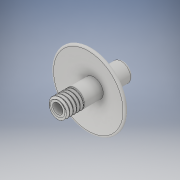
# Autodesk Inventor part: Kabelzugentlastung
Saved by Autodesk Inventor 2018.2 (Build 222227000, 227)
## iProperties
Created: 2018-01-25
Part Number: Kabelzugentlastung
Material: Generisch
Document SubType Name: Modeling
Designer: JochenAlt
Density: 1 g/cm^3
Appearance: Vorgabe
Author: JochenAlt
Autodesk Inventor part; units mm, degrees
ref_plane "YZ Plane" through (0, 0, 0) normal (1, 0, 0) x (0, 1, 0)
ref_plane "XZ Plane" through (0, 0, 0) normal (0, 1, 0) x (-1, 0, 0)
ref_plane "XY Plane" through (0, 0, 0) normal (0, 0, 1) x (1, 0, 0)
sketch "Skizze1" plane through (0, 0, 0) normal (0, 0, 1) x (1, 0, 0)
  line L0 (0, 93.8392) -> (0, -15.6399) construction
  line L1 (-4.2899, 0) -> (25.7393, 0) construction
  arc A0 (20.2057, 57.5563) -> (5.5, 60.7515) centre (0, 0) ccw
  arc A1 (20.09, 59.1831) -> (6.1759, 62.1941) centre (0, 0) ccw
  arc A2 (20.2057, 57.5563) -> (20.09, 59.1831) centre (20.5, 58.3948) ccw
  line L2 (5.5, 62.9404) -> (5.5, 76.6904)
  line L3 (4.25, 77.9404) -> (4.25, 77.9404)
  arc A3 (5.5, 62.9404) -> (6.1759, 62.1941) centre (6.25, 62.9404) ccw
  arc A4 (5.5, 76.6904) -> (4.25, 77.9404) centre (4.25, 76.6904) ccw
  arc A5 (4.25, 77.9404) -> (3, 76.6904) centre (4.25, 76.6904) ccw
  line L4 (5.5, 60.7515) -> (5.5, 39.7947)
  line L5 (3, 76.6904) -> (3, 62.9881)
  line L6 (3, 62.9881) -> (3, 39.7947)
  line L7 (3, 39.7947) -> (5.5, 39.7947)
  point P0 (20.0791, 59.1868)
  point P1 (17.7943, 58.3469)
  point P2 (20.1696, 59.2201)
  point P3 (20.1696, 59.2201)
  point P4 (5.5, 62.2575)
  dimension "d3" = 1.5
  dimension "d4" = 61
  dimension "d6" = 5.5
  dimension "d9" = 0.75
  dimension "d10" = 15
  dimension "d11" = 1.25
  dimension "d59" = 2.5
  dimension "d60" = 15
  constraints: 16 point on circle, 12 end point, 7 tangent, 6 centre point, 3 coincident, 2 vertical, 1 collinear, 1 concentric, 1 horizontal, 1 perpendicular, 1 point on line, 5 other
  measures "d3" radial gap between concentric circles of A1 A0
  measures "d4" radius of A0
  measures "d6" distance between parallel lines of L2 L0
  measures "d9" radius of A3
  measures "d10" distance from line of A3.centre L3
  measures "d11" radius of A4
  measures "d59" distance of L4.end L6.end
  measures "d60" horizontal distance of A2.centre L2.start
revolve "Umdrehung1" add sketch "Skizze1" angle 360 about axis through (0, 0, 0) along (0, -1, 0)
thread "Gewinde3" size "TR11x2" class "7e" standard "ISO Metric Trapezoidal Threads" length 10
sketch "Skizze12" plane through (0, 39.7947, 0) normal (-1, 0, 0) x (0, 0, 1)
  line L0 (5.5, 0) -> (5.5, 10)
  line L1 (5.5, 10) -> (4.1948, 10)
  line L2 (4.1948, 10) -> (4.1948, 0)
  line L3 (4.1948, 0) -> (5.5, 0)
  line L4 (0, -10.2682) -> (0, 46.2147) projected
  constraints: 8 end point
revolve "Umdrehung8" cut sketch "Skizze12" angle 360 about axis through (0, 39.7947, 0) along (0, 1, 0)
sketch "Skizze13" plane through (0, 39.7947, 0) normal (-1, 0, 0) x (0, 0, 1)
  line L0 (5.5, 0) -> (5.5, 10)
  line L1 (5.5, 10) -> (4.1948, 10)
  line L2 (4.1948, 10) -> (4.1948, 0)
  line L3 (4.1948, 0) -> (5.5, 0)
  line L4 (0, -10.2682) -> (0, 46.2147) projected
  constraints: 8 end point
revolve "Umdrehung9" add sketch "Skizze13" angle 360 about axis through (0, 39.7947, 0) along (0, 1, 0) separate body
sketch "Skizze11" plane through (0, 39.7947, 0) normal (1, 0, 0) x (0, 1, 0)
  line L0 (-1.1849, -4.3017) -> (-1.0001, -4.3017) construction
  line L1 (0.1847, -5.3934) -> (-0.0001, -5.7136) construction
  line L2 (-2.0001, -5.7136) -> (-2.185, -5.3934) construction
  line L3 (-0.8153, -4.3017) -> (-1.0001, -3.9816) construction
  line L4 (-1.0001, -3.9816) -> (-1.1849, -4.3017) construction
  line L5 (-2.0001, -5.7136) -> (-1.8153, -5.3934) construction
  line L6 (-0.8153, -4.3017) -> (-0.1849, -5.3934)
  line L7 (-2.185, -5.3934) -> (-1.8153, -5.3934) construction
  arc A0 (-2.185, -5.3934) -> (-2.0001, -5.5002) centre (-2.0001, -5.2867) ccw construction
  line L8 (0.1847, -5.3934) -> (-0.1849, -5.3934) construction
  line L9 (-2.0001, -5.7136) -> (-2.0001, -5.3934) construction
  line L10 (-0.0001, -5.7136) -> (-0.0001, -5.3934) construction
  line L11 (-1.0001, -3.9816) -> (-1.0001, -4.195) construction
  line L12 (-2.0001, -5.5002) -> (-0.0001, -5.5002)
  arc A1 (-2.0001, -5.5002) -> (-1.8153, -5.3934) centre (-2.0001, -5.2867) ccw
  line L13 (-0.1849, -5.3934) -> (-0.0001, -5.7136) construction
  line L14 (-1.8153, -5.3934) -> (-1.1849, -4.3017)
  line L15 (-0.0001, -0.0002) -> (-0.0001, 0.0177)
  line L16 (-0.0001, 0.0177) -> (-0.0001, -0.0002)
  line L17 (-0.0001, -0.0002) -> (0.0334, -0.0002)
  arc A2 (-0.1849, -5.3934) -> (-0.0001, -5.5002) centre (-0.0001, -5.2867) ccw
  arc A3 (-0.0001, -5.5002) -> (0.1847, -5.3934) centre (-0.0001, -5.2867) ccw construction
  arc A4 (-1.0001, -4.195) -> (-1.1849, -4.3017) centre (-1.0001, -4.4084) ccw
  arc A5 (-0.8153, -4.3017) -> (-1.0001, -4.195) centre (-1.0001, -4.4084) ccw
  line L18 (-1.0001, -4.195) -> (-1.0001, -4.3017) construction
  line L19 (-1.0001, -4.3017) -> (-0.8153, -4.3017) construction
  dimension "d83" = 60
  dimension "d84" = 0.3202
  dimension "d85" = 0.3202
  dimension "Skizze11_ThreadOffset" = 0
  dimension "Skizze11_MajorRadius" = 5.5
  dimension "d88" = 2
  dimension "Skizze11_MinorRadius" = 4.1948
  constraints: 40 end point, 12 point on circle, 10 parallel, 8 tangent, 6 centre point, 6 collinear, 2 midpoint, 2 point on line, 1 horizontal, 1 perpendicular, 3 other
  measures "d83" angle of L6 L14
  measures "d84" distance of L3.end L0.end
  measures "d85" distance of L1.end L10.end
  measures "Skizze11_ThreadOffset" distance between parallel lines of L15 L10
  measures "Skizze11_MajorRadius" distance from line of L12 L15.start
  measures "d88" distance from line of L1.end L9
  measures "Skizze11_MinorRadius" distance edge to line of A5 L17
coil "Spirale4" sketch "Skizze11" operation cut axis through (0, 39.7947, 0) along (0, 1, 0) pitch 2.002 turns 6.993007 hand right bodies 2
equation "\"d9\" = 0.5 * d3"
equation "\"d10\" = d16"
equation "\"d11\" = 0.5 * d59"
equation "\"d83\" = d90"
equation "\"d84\" = 0.160083 * Skizze11_Pitch"
equation "\"d85\" = 0.160083 * Skizze11_Pitch"
equation "\"d88\" = Skizze11_Pitch"
equation "\"d26\" = 60deg"
equation "\"Skizze2_Pitch\" = 1"
equation "\"d47\" = 60deg"
equation "\"Skizze5_Pitch\" = 2"
equation "\"d70\" = 60deg"
equation "\"Skizze8_Pitch\" = 2"
equation "\"d90\" = 60deg"
equation "\"Skizze11_Pitch\" = 2"
equation "\"d16\" = 15"
